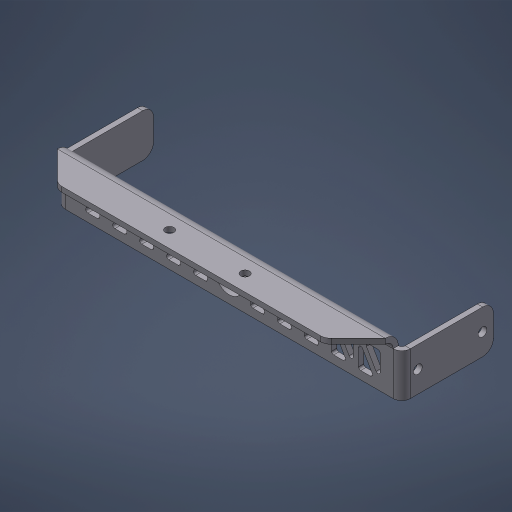
# Autodesk Inventor part: PLATE,SUPPORT,STOP,ARM
Saved by Autodesk Inventor 2024.3 (Build 283343000, 343)
## iProperties
Category: _
Manager: _
Created: 2025-03-17
Part Number: PLATE,SUPPORT,STOP,ARM
Checked By: 00
Engr Approved By: _
User Status: Work In Process
Material: Aluminum, 355-T6
Description: SHEET METAL (mm)
Document SubType Name: Sheet Metal
Mfg Approved By: John.Thibert
Designer: John.Thibert
Manufacturer: Standard
Standards Organization: Custom
Mass: 90.599 g
Surface Area: 264.79 cm^2
Volume: 33.4314 cm^3
Density: 2.71 g/cm^3
Sheet Metal Rule: Default
Appearance: Metal-AL-6061 (Flat)
Flat Pattern Width: 5.24683 cm
Flat Pattern Length: 30.1427 cm
Flat Pattern Area: 158.154 cm^2
Sheet Metal Width: 2.066 in
Sheet Metal Length: 11.867 in
Sheet Metal Area: 24.514 in^2
CN_MASS: 0.09
CL_runCount: 1
CN_SERVICEABLE: _
FIRST_DESCRIPTION: _
SECOND_DESCRIPTION: _
THIRD_DESCRIPTION: _
ModelCat: Uncategorized
MaterialName: Aluminum, 355-T6
ILogicPurgeVersion: 2.2.20.20
OnSaveVersion: 3.5.0.0
OnSaveAssembly: COREAutomationManager
Subject: _
Author: John.Thibert
Keywords: -
Revision Number: A
Autodesk Inventor part; units mm, degrees
ref_plane "YZ Plane" through (0, 0, 0) normal (1, 0, 0) x (0, 1, 0)
ref_plane "XZ Plane" through (0, 0, 0) normal (0, 1, 0) x (-1, 0, 0)
ref_plane "XY Plane" through (0, 0, 0) normal (0, 0, 1) x (1, 0, 0)
sketch "Sketch1" plane through (0, 0, 0) normal (0, 0, 1) x (1, 0, 0)
  line L0 (-101.6, 12.7) -> (101.6, 12.7)
  line L1 (101.6, 12.7) -> (101.6, -12.7)
  line L2 (101.6, -12.7) -> (-101.6, -12.7)
  line L3 (-101.6, -12.7) -> (-101.6, 12.7)
  line L4 (-101.6, 12.7) -> (101.6, -12.7) construction
  line L5 (101.6, 12.7) -> (-101.6, -12.7) construction
  point P0 (0, 0)
  dimension "d0" = 203.2
  dimension "d1" = 25.4
  measures "d0" distance of L1.end L2.end
  measures "d1" distance of L0.end L1.end
extrude "Plate1" add sketch "Sketch1" along normal blind 3.048
sketch "Sketch8" plane through (98.552, -12.7, 3.048) normal (1, 0, 0) x (0, 1, 0)
  line L0 (25.4, 0) -> (0, 0)
  line L1 (0, 0) -> (0, -53.975)
  line L2 (0, -53.975) -> (25.4, -53.975)
  line L3 (25.4, -53.975) -> (25.4, 0)
  constraints: 6 end point, 1 horizontal, 1 perpendicular, 1 vertical
edge flange "Flange2" height 53.975 angle 90 thickness 3.048 bend radius 2.032 thickness toward (1, 0, 0) relief tear relief width 3.048 relief depth 1.524 corner gap 4.572 corner form 0 edges at (101.6, 0, 0) (-101.6, 0, 0) wall of the first edge with corners at (98.552, 12.7, 3.048) (98.552, -12.7, 3.048) (98.552, -12.7, -50.927) (98.552, 12.7, -50.927)
bend "Bend2"
corner "Corner2"
sketch "Sketch2" plane through (-96.52, 17.272, 7.62) normal (0, 1, 0) x (-1, 0, 0)
  line L0 (-193.04, 0) -> (0, 0)
  line L1 (0, 0) -> (0, 17.78)
  line L2 (0, 17.78) -> (-193.04, 17.78)
  line L3 (-193.04, 17.78) -> (-193.04, 0)
  constraints: 6 end point, 1 horizontal, 1 perpendicular, 1 vertical
edge flange "Flange1" height 25.4 angle 90 thickness 3.048 bend radius 4.572 thickness toward (0, 1, 0) relief tear relief width 3.048 relief depth 1.524 edges at (0, 12.7, 3.048) wall of the first edge with corners at (96.52, 17.272, 7.62) (-96.52, 17.272, 7.62) (-96.52, 17.272, 25.4) (96.52, 17.272, 25.4)
bend "Bend1"
corner "Corner1"
chamfer "Corner Chamfer1" distance 17.78 angle 45 2 edges at (96.52, 18.796, 25.4) (-96.52, 18.796, 25.4)
fillet "Corner Round1" radius 6.35 6 edges at (78.74, 18.796, 25.4) (-78.74, 18.796, 25.4) (-100.076, -12.7, -50.927) (-100.076, 12.7, -50.927) (100.076, 12.7, -50.927) (100.076, -12.7, -50.927)
sketch "Sketch5" plane through (0, 0, 3.048) normal (0, 0, 1) x (1, 0, 0)
  line L0 (12.7, -7.9375) -> (12.7, 7.9375)
  line L1 (12.7, 7.9375) -> (21.8654, -7.9375)
  line L2 (21.8654, -7.9375) -> (12.7, -7.9375)
  line L3 (25.4, -7.9375) -> (16.2346, 7.9375)
  line L4 (16.2346, 7.9375) -> (25.4, 7.9375)
  line L5 (25.4, 7.9375) -> (25.4, -7.9375)
  line L6 (-142.24, 0) -> (142.24, 0) construction
  point P0 (0, 0)
  point P1 (12.7, 0)
  dimension "d36" = 12.7
  dimension "d37" = 15.875
  dimension "d38" = 60
  dimension "d39" = 12.7
  constraints: 12 end point, 3 point on line, 2 parallel, 2 perpendicular, 1 midpoint, 1 vertical
  measures "d36" distance between parallel lines of L0 L5
  measures "d37" distance of L0.start L0.end
  measures "d38" angle of L2 L1
  measures "d39" distance from line of point (0, 0) L0
extrude "Cut1" cut sketch "Sketch5" against normal blind 3.048
fillet "Corner Round2" radius 1.27 6 edges at (25.4, 7.9375, 1.524) (25.4, -7.9375, 1.524) (16.2346, 7.9375, 1.524) (21.8654, -7.9375, 1.524) (12.7, -7.9375, 1.524) (12.7, 7.9375, 1.524)
pattern_linear "Rectangular Pattern2" count 5 spacing 15.875 along (1, 0, 0) of "Cut1", "Corner Round2"
mirror "Mirror1" about plane through (0, 0, 0) normal (1, 0, 0) of "Cut1", "Corner Round2", "Rectangular Pattern2"
sketch "Sketch6" plane through (0, 0, 3.048) normal (0, 0, 1) x (1, 0, 0)
  circle A0 centre (0, 0) radius 6 construction
  dimension "d46" = 12
  constraints: 2 coincident, 1 centre point
  measures "d46" diameter of A0
hole "Hole3" at (0, 0, 3.048) direction (0, 0, -1) diameter 16 end through all
sketch "Sketch7" plane through (-96.52, 17.272, 7.62) normal (0, -1, 0) x (1, 0, 0)
  line L0 (172.6297, 17.78) -> (20.4103, 17.78) construction
  line L1 (118.745, 8.255) -> (74.295, 8.255) construction
  line L2 (96.52, 33.0454) -> (96.52, -73.8124) construction
  point P0 (96.52, -7.62)
  point P1 (96.52, 8.255)
  dimension "d55" = 44.45
  dimension "d56" = 9.525
  constraints: 2 end point, 1 horizontal, 1 midpoint, 1 point on line
  measures "d55" distance of L1.start L1.end
  measures "d56" distance between parallel lines of L1 L0
hole "Hole4" at (22.225, 17.272, 15.875) at (-22.225, 17.272, 15.875) direction (0, 1, 0) diameter 5.1054 end through all clearance for "Flat Head Machine Screw (82)" size "#10" standard "Ansi Unified Screw Threads"
sketch "Sketch9" plane through (98.552, -12.7, -2.032) normal (-1, 0, 0) x (0, 0, 1)
  line L0 (-4.445, 12.7) -> (-42.545, 12.7) construction
  line L1 (2.032, 30.48) -> (2.032, -5.08) construction
  line L2 (-48.895, 19.05) -> (-48.895, 6.35) construction
  point P0 (2.032, 12.7)
  dimension "d74" = 6.35
  dimension "d75" = 38.1
  constraints: 2 end point, 1 horizontal, 1 point on line
  measures "d74" distance from line of L0.end L2
  measures "d75" distance of L0.start L0.end
hole "Hole5" at (98.552, 0, -44.577) at (98.552, 0, -6.477) direction (1, 0, 0) diameter 5.1054 end through all clearance for "Flat Head Machine Screw (82)" size "#10" standard "Ansi Unified Screw Threads"
equation "\"d40\" = Thickness"
equation "\"d2\" = Thickness"
equation "\"d3\" = BendReliefWidth"
equation "\"d4\" = BendReliefDepth"
equation "\"d5\" = MinimumRemnant"
equation "\"d6\" = TransitionRadius"
equation "\"d9\" = BendRadius"
equation "\"d10\" = CornerReliefSize"
equation "\"d11\" = GapSize"
equation "\"d12\" = JacobiRadiusSize"
equation "\"d64\" = BendReliefWidth"
equation "\"d65\" = BendReliefDepth"
equation "\"d66\" = MinimumRemnant"
equation "\"d67\" = TransitionRadius"
equation "\"d71\" = CornerReliefSize"
equation "\"d72\" = GapSize"
equation "\"d73\" = JacobiRadiusSize"
equation "\"BendRadius\" = 1.5 * Thickness"
equation "\"BendReliefWidth\" = Thickness"
equation "\"BendReliefDepth\" = 0.5 * Thickness"
equation "\"CornerReliefSize\" = 4 * Thickness"
equation "\"MinimumRemnant\" = 2 * Thickness"
equation "\"TransitionRadius\" = BendRadius"
equation "\"JacobiRadiusSize\" = BendRadius"
equation "\"GapSize\" = Thickness"
equation "\"Thickness\" = 3.048"
body "Solid1"
